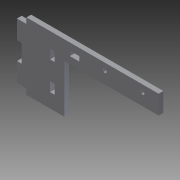
# Autodesk Inventor part: side 2
Saved by Autodesk Inventor 2011 (Build 150239000, 239)
## iProperties
Created: 2011-02-20
Part Number: side 2
Document SubType Name: Modeling
Designer: adowning
Density: 1 g/cm^3
Author: adowning
Autodesk Inventor part; units mm, degrees
ref_plane "YZ Plane" through (0, 0, 0) normal (1, 0, 0) x (0, 1, 0)
ref_plane "XZ Plane" through (0, 0, 0) normal (0, 1, 0) x (-1, 0, 0)
ref_plane "XY Plane" through (0, 0, 0) normal (0, 0, 1) x (1, 0, 0)
sketch "Sketch2" plane through (0, 0, 0) normal (0, 0, 1) x (1, 0, 0)
  line L0 (-75.3899, 25.3495) -> (108.7601, 25.3495)
  line L1 (108.7601, 25.3495) -> (108.7601, -0.0505)
  line L2 (108.7601, -0.0505) -> (-18.2399, -0.0505)
  line L3 (-75.3899, 25.3495) -> (-75.3899, -64.8205)
  line L4 (-75.3899, -64.8205) -> (-18.2399, -64.8205)
  line L5 (-18.2399, -64.8205) -> (-18.2399, -0.0505)
  line L6 (-75.3899, 25.3495) -> (-81.7399, 25.3495)
  line L7 (-81.7399, 25.3495) -> (-81.7399, -0.0505)
  line L8 (-81.7399, -0.0505) -> (-75.3899, -0.0505)
  line L9 (-75.3899, -64.8205) -> (-81.7399, -64.8205)
  line L10 (-81.7399, -64.8205) -> (-81.7399, -39.4205)
  line L11 (-81.7399, -39.4205) -> (-75.3899, -39.4205)
  line L12 (108.7601, 25.3495) -> (87.1701, 25.3495)
  line L13 (87.1701, 25.3495) -> (87.1701, 15.8245)
  line L14 (87.1701, 15.8245) -> (36.3701, 15.8245)
  circle A0 centre (36.3701, 15.8245) radius 2.4892
  circle A1 centre (87.1701, 15.8245) radius 2.4892
  line L15 (-18.2399, -64.8205) -> (-18.2399, -45.7705)
  line L16 (-18.2399, -45.7705) -> (-37.2899, -45.7705)
  line L17 (-37.2899, -45.7705) -> (-37.2899, -33.0705)
  line L18 (-37.2899, -33.0705) -> (-30.9399, -33.0705)
  line L19 (-30.9399, -33.0705) -> (-30.9399, -7.6705)
  line L20 (-30.9399, -7.6705) -> (-37.2899, -7.6705)
  line L21 (-37.2899, -7.6705) -> (-37.2899, 5.0295)
  line L22 (-37.2899, 5.0295) -> (-30.9399, 5.0295)
  line L23 (-30.9399, 5.0295) -> (-30.9399, -7.6705)
  line L24 (-30.9399, -33.0705) -> (-30.9399, -45.7705)
  point P0 (0, 0)
  dimension "d5" = 184.15
  dimension "d6" = 25.4
  dimension "d7" = 127
  dimension "d8" = 90.17
  dimension "d9" = 6.35
  dimension "d10" = 25.4
  dimension "d11" = 25.4
  dimension "d12" = 21.59
  dimension "d13" = 9.525
  dimension "d14" = 50.8
  dimension "d15" = 4.9784
  dimension "d16" = 4.9784
  dimension "d17" = 19.05
  dimension "d18" = 19.05
  dimension "d19" = 12.7
  dimension "d20" = 6.35
  dimension "d21" = 25.4
  dimension "d22" = 6.35
  dimension "d23" = 12.7
  constraints: 50 end point, 13 perpendicular, 8 parallel, 5 point on line, 2 centre point, 2 coincident, 1 collinear, 1 horizontal
  measures "d5" distance of L0.start L0.end
  measures "d6" distance of L0.end L1.end
  measures "d7" distance of L1.end L2.end
  measures "d8" distance of L0.start L3.end
  measures "d9" distance of L0.start L6.end
  measures "d10" distance of L6.end L7.end
  measures "d11" distance of L9.end L10.end
  measures "d12" distance of L0.end L12.end
  measures "d13" distance of L12.end L13.end
  measures "d14" distance of L13.end L14.end
  measures "d15" diameter of A0
  measures "d16" diameter of A1
  measures "d17" distance of L4.end L15.end
  measures "d18" distance of L15.end L16.end
  measures "d19" distance of L16.end L17.end
  measures "d20" distance of L17.end L18.end
  measures "d21" distance of L18.end L19.end
  measures "d22" distance of L19.end L20.end
  measures "d23" distance of L20.end L21.end
extrude "Extrusion1" add sketch "Sketch2" along normal blind 6.35
sketch "Sketch3" plane through (0, 0, 6.35) normal (0, 0, 1) x (1, 0, 0)
  line L0 (-81.7399, 25.3495) -> (108.7601, 25.3495) projected
  line L1 (-81.7399, -0.0505) -> (-81.7399, 25.3495) projected
  line L2 (-75.3899, -0.0505) -> (-81.7399, -0.0505) projected
  line L3 (-81.7399, -39.4205) -> (-75.3899, -39.4205) projected
  line L4 (-81.7399, -64.8205) -> (-81.7399, -39.4205) projected
  line L5 (-18.2399, -64.8205) -> (-81.7399, -64.8205) projected
  line L6 (-75.3899, -0.0505) -> (-75.3899, 12.6495)
  line L7 (-75.3899, 12.6495) -> (-69.0399, 12.6495)
  line L8 (-69.0399, 12.6495) -> (-69.0399, 25.3495)
  line L9 (-75.3899, -39.4205) -> (-75.3899, -52.1205)
  line L10 (-75.3899, -52.1205) -> (-69.0399, -52.1205)
  line L11 (-69.0399, -52.1205) -> (-69.0399, -64.8205)
  point P0 (0, 0)
  dimension "d26" = 12.7
  dimension "d27" = 6.35
  dimension "d28" = 12.7
  dimension "d29" = 6.35
  constraints: 12 end point, 5 perpendicular, 2 point on line, 1 parallel
  measures "d26" distance of L2.start L6.end
  measures "d27" distance of L6.end L7.end
  measures "d28" distance of L3.end L9.end
  measures "d29" distance of L9.end L10.end
extrude "Extrusion2" cut sketch "Sketch3" against normal blind 25.4
sketch "Sketch4" plane through (0, 0, 6.35) normal (0, 0, 1) x (1, 0, 0)
  line L0 (-75.3899, 12.6495) -> (-75.3899, -52.1205) projected
  line L1 (-75.3899, -52.1205) -> (-69.0399, -52.1205) projected
  line L2 (-69.0399, -52.1205) -> (-69.0399, -64.8205) projected
  line L3 (-69.0399, 25.3495) -> (-69.0399, 12.6495) projected
  line L4 (-69.0399, 12.6495) -> (-75.3899, 12.6495) projected
  line L5 (-69.0399, 25.3495) -> (-69.0399, 17.7295)
  line L6 (-69.0399, 17.7295) -> (-81.7399, 17.7295)
  line L7 (-81.7399, 17.7295) -> (-81.7399, -7.6705)
  line L8 (-81.7399, -7.6705) -> (-75.3899, -7.6705)
  line L9 (-69.0399, -64.8205) -> (-69.0399, -57.2005)
  line L10 (-69.0399, -57.2005) -> (-81.7399, -57.2005)
  line L11 (-81.7399, -57.2005) -> (-81.7399, -31.8005)
  line L12 (-81.7399, -31.8005) -> (-75.3899, -31.8005)
  point P0 (0, 0)
  dimension "d32" = 7.62
  dimension "d33" = 12.7
  dimension "d34" = 25.4
  dimension "d35" = 7.62
  dimension "d36" = 12.7
  dimension "d37" = 25.4
  constraints: 16 end point, 4 perpendicular, 4 point on line, 2 parallel
  measures "d32" distance of L3.start L5.end
  measures "d33" distance of L5.end L6.end
  measures "d34" distance of L6.end L7.end
  measures "d35" distance of L2.end L9.end
  measures "d36" distance of L9.end L10.end
  measures "d37" distance of L10.end L11.end
extrude "Extrusion3" add sketch "Sketch4" against normal blind 25.4
sketch "Sketch5" plane through (0, 0, 6.35) normal (0, 0, 1) x (1, 0, 0)
  line L0 (-81.7399, -57.2005) -> (-69.0399, -57.2005) projected
  line L1 (-69.0399, 17.7295) -> (-81.7399, 17.7295) projected
  line L2 (-30.9399, -33.0705) -> (-30.9399, -45.7705) projected
  line L3 (-69.0399, 17.7295) -> (-69.0399, 15.1895)
  line L4 (-69.0399, 15.1895) -> (-75.3899, 15.1895)
  line L5 (-75.3899, 15.1895) -> (-75.3899, 17.7295)
  line L6 (-69.0399, -57.2005) -> (-69.0399, -54.6605)
  line L7 (-69.0399, -54.6605) -> (-75.3899, -54.6605)
  line L8 (-75.3899, -54.6605) -> (-75.3899, -57.2005)
  point P0 (0, 0)
  dimension "d40" = 2.54
  dimension "d41" = 2.54
  constraints: 12 end point, 3 parallel, 2 midpoint, 1 perpendicular
  measures "d40" distance of L1.start L3.end
  measures "d41" distance of L0.end L6.end
extrude "Extrusion4" cut sketch "Sketch5" against normal blind 25.4
sketch "Sketch6" plane through (-81.7399, -7.6705, 6.35) normal (-1, 0, 0) x (0, 0, 1)
  line L0 (0, 25.4) -> (-25.4, 25.4) projected
  line L1 (0, 25.4) -> (-6.35, 25.4)
  line L2 (-6.35, 25.4) -> (-6.35, -76.2)
  line L3 (-6.35, -76.2) -> (-39.1891, -38.2837)
  line L4 (-39.1891, -38.2837) -> (-39.1891, 49.1671)
  line L5 (-39.1891, 49.1671) -> (-6.35, 49.1671)
  line L6 (-6.35, 49.1671) -> (-6.35, 25.4)
  point P0 (-6.35, 7.6705)
  dimension "d44" = 101.6
  constraints: 12 end point, 2 perpendicular, 1 collinear, 1 parallel, 1 point on line
  measures "d44" distance of L1.end L2.end
extrude "Extrusion5" cut sketch "Sketch6" against normal blind 25.4
sketch "Sketch7" plane through (0, 0, 6.35) normal (0, 0, 1) x (1, 0, 0)
  line L0 (-75.3899, 15.1895) -> (-75.3899, 17.7295) projected
  line L1 (-75.3899, -57.2005) -> (-75.3899, -54.6605) projected
  line L2 (-75.3899, -54.6605) -> (-69.0399, -54.6605) projected
  line L3 (-69.0399, -54.6605) -> (-69.0399, -64.8205) projected
  line L4 (-69.0399, 25.3495) -> (-69.0399, 15.1895) projected
  line L5 (-69.0399, 15.1895) -> (-75.3899, 15.1895) projected
  line L6 (-75.3899, 17.7295) -> (-69.0399, 17.7295)
  line L7 (-75.3899, -57.2005) -> (-69.0399, -57.2005)
  point P0 (0, 0)
  constraints: 4 end point, 2 perpendicular, 2 point on line
extrude "Extrusion6" add sketch "Sketch7" against normal blind 6.35
sketch "Sketch8" plane through (0, 0, 6.35) normal (0, 0, 1) x (1, 0, 0)
  line L0 (108.7601, -0.0505) -> (-18.2399, -0.0505) projected
  line L1 (-69.0399, 25.3495) -> (108.7601, 25.3495) projected
  line L2 (108.7601, 25.3495) -> (14.7801, 25.3495)
  line L3 (14.7801, 25.3495) -> (14.7801, 9.4745)
  line L4 (14.7801, 9.4745) -> (14.7801, 15.8245)
  line L5 (14.7801, 15.8245) -> (2.0801, 15.8245)
  line L6 (2.0801, 15.8245) -> (2.0801, 9.4745)
  line L7 (2.0801, 9.4745) -> (-10.6199, 9.4745)
  line L8 (-10.6199, 9.4745) -> (-10.6199, 15.8245)
  line L9 (-10.6199, 15.8245) -> (2.0801, 15.8245)
  point P0 (0, 0)
  dimension "d49" = 93.98
  dimension "d50" = 15.875
  dimension "d51" = 6.35
  dimension "d52" = 12.7
  dimension "d53" = 12.7
  constraints: 16 end point, 4 perpendicular, 2 point on line, 1 collinear, 1 parallel
  measures "d49" distance of L1.end L2.end
  measures "d50" distance of L2.end L3.end
  measures "d51" distance of L3.end L4.end
  measures "d52" distance of L4.end L5.end
  measures "d53" distance of L6.end L7.end
extrude "Extrusion7" cut sketch "Sketch8" against normal blind 25.4
body "Solid1"
